Autodesk Inventor part; units mm, degrees
(part 4 of 4)
  line L912 (65.6705, -8.3885) -> (64.6705, -6.6564) projected
  line L913 (64.6705, -6.6564) -> (65.6705, -4.9244) projected
  line L914 (65.6705, -4.9244) -> (67.6705, -4.9244) projected
  line L915 (67.6705, -4.9244) -> (68.6705, -6.6564) projected
  line L916 (68.6705, -6.6564) -> (67.6705, -8.3885) projected
  line L917 (67.6705, -8.3885) -> (65.6705, -8.3885) projected
  line L918 (60.9385, -5.6564) -> (59.9385, -3.9244) projected
  line L919 (59.9385, -3.9244) -> (60.9385, -2.1923) projected
  line L920 (60.9385, -2.1923) -> (62.9385, -2.1923) projected
  line L921 (62.9385, -2.1923) -> (63.9385, -3.9244) projected
  line L922 (63.9385, -3.9244) -> (62.9385, -5.6564) projected
  line L923 (62.9385, -5.6564) -> (60.9385, -5.6564) projected
  line L924 (56.2064, -8.3885) -> (55.2064, -6.6564) projected
  line L925 (55.2064, -6.6564) -> (56.2064, -4.9244) projected
  line L926 (56.2064, -4.9244) -> (58.2064, -4.9244) projected
  line L927 (58.2064, -4.9244) -> (59.2064, -6.6564) projected
  line L928 (59.2064, -6.6564) -> (58.2064, -8.3885) projected
  line L929 (58.2064, -8.3885) -> (56.2064, -8.3885) projected
  line L930 (51.4744, -5.6564) -> (50.4744, -3.9244) projected
  line L931 (50.4744, -3.9244) -> (51.4744, -2.1923) projected
  line L932 (51.4744, -2.1923) -> (53.4744, -2.1923) projected
  line L933 (53.4744, -2.1923) -> (54.4744, -3.9244) projected
  line L934 (54.4744, -3.9244) -> (53.4744, -5.6564) projected
  line L935 (53.4744, -5.6564) -> (51.4744, -5.6564) projected
  line L936 (46.7423, -8.3885) -> (45.7423, -6.6564) projected
  line L937 (45.7423, -6.6564) -> (46.7423, -4.9244) projected
  line L938 (46.7423, -4.9244) -> (48.7423, -4.9244) projected
  line L939 (48.7423, -4.9244) -> (49.7423, -6.6564) projected
  line L940 (49.7423, -6.6564) -> (48.7423, -8.3885) projected
  line L941 (48.7423, -8.3885) -> (46.7423, -8.3885) projected
  line L942 (42.0103, -5.6564) -> (41.0103, -3.9244) projected
  line L943 (41.0103, -3.9244) -> (42.0103, -2.1923) projected
  line L944 (42.0103, -2.1923) -> (44.0103, -2.1923) projected
  line L945 (44.0103, -2.1923) -> (45.0103, -3.9244) projected
  line L946 (45.0103, -3.9244) -> (44.0103, -5.6564) projected
  line L947 (44.0103, -5.6564) -> (42.0103, -5.6564) projected
  line L948 (37.2782, -8.3885) -> (36.2782, -6.6564) projected
  line L949 (36.2782, -6.6564) -> (37.2782, -4.9244) projected
  line L950 (37.2782, -4.9244) -> (39.2782, -4.9244) projected
  line L951 (39.2782, -4.9244) -> (40.2782, -6.6564) projected
  line L952 (40.2782, -6.6564) -> (39.2782, -8.3885) projected
  line L953 (39.2782, -8.3885) -> (37.2782, -8.3885) projected
  line L954 (32.5462, -5.6564) -> (31.5462, -3.9244) projected
  line L955 (31.5462, -3.9244) -> (32.5462, -2.1923) projected
  line L956 (32.5462, -2.1923) -> (34.5462, -2.1923) projected
  line L957 (34.5462, -2.1923) -> (35.5462, -3.9244) projected
  line L958 (35.5462, -3.9244) -> (34.5462, -5.6564) projected
  line L959 (34.5462, -5.6564) -> (32.5462, -5.6564) projected
  line L960 (27.8141, -8.3885) -> (26.8141, -6.6564) projected
  line L961 (26.8141, -6.6564) -> (27.8141, -4.9244) projected
  line L962 (27.8141, -4.9244) -> (29.8141, -4.9244) projected
  line L963 (29.8141, -4.9244) -> (30.8141, -6.6564) projected
  line L964 (30.8141, -6.6564) -> (29.8141, -8.3885) projected
  line L965 (29.8141, -8.3885) -> (27.8141, -8.3885) projected
  line L966 (23.0821, -5.6564) -> (22.0821, -3.9244) projected
  line L967 (22.0821, -3.9244) -> (23.0821, -2.1923) projected
  line L968 (23.0821, -2.1923) -> (25.0821, -2.1923) projected
  line L969 (25.0821, -2.1923) -> (26.0821, -3.9244) projected
  line L970 (26.0821, -3.9244) -> (25.0821, -5.6564) projected
  line L971 (25.0821, -5.6564) -> (23.0821, -5.6564) projected
  line L972 (75.1346, -2.9244) -> (74.1346, -1.1923) projected
  line L973 (74.1346, -1.1923) -> (75.1346, 0.5397) projected
  line L974 (75.1346, 0.5397) -> (77.1346, 0.5397) projected
  line L975 (77.1346, 0.5397) -> (78.1346, -1.1923) projected
  line L976 (78.1346, -1.1923) -> (77.1346, -2.9244) projected
  line L977 (77.1346, -2.9244) -> (75.1346, -2.9244) projected
  line L978 (70.4026, -0.1923) -> (69.4026, 1.5397) projected
  line L979 (69.4026, 1.5397) -> (70.4026, 3.2718) projected
  line L980 (70.4026, 3.2718) -> (72.4026, 3.2718) projected
  line L981 (72.4026, 3.2718) -> (73.4026, 1.5397) projected
  line L982 (73.4026, 1.5397) -> (72.4026, -0.1923) projected
  line L983 (72.4026, -0.1923) -> (70.4026, -0.1923) projected
  line L984 (65.6705, -2.9244) -> (64.6705, -1.1923) projected
  line L985 (64.6705, -1.1923) -> (65.6705, 0.5397) projected
  line L986 (65.6705, 0.5397) -> (67.6705, 0.5397) projected
  line L987 (67.6705, 0.5397) -> (68.6705, -1.1923) projected
  line L988 (68.6705, -1.1923) -> (67.6705, -2.9244) projected
  line L989 (67.6705, -2.9244) -> (65.6705, -2.9244) projected
  line L990 (60.9385, -0.1923) -> (59.9385, 1.5397) projected
  line L991 (59.9385, 1.5397) -> (60.9385, 3.2718) projected
  line L992 (60.9385, 3.2718) -> (62.9385, 3.2718) projected
  line L993 (62.9385, 3.2718) -> (63.9385, 1.5397) projected
  line L994 (63.9385, 1.5397) -> (62.9385, -0.1923) projected
  line L995 (62.9385, -0.1923) -> (60.9385, -0.1923) projected
  line L996 (56.2064, -2.9244) -> (55.2064, -1.1923) projected
  line L997 (55.2064, -1.1923) -> (56.2064, 0.5397) projected
  line L998 (56.2064, 0.5397) -> (58.2064, 0.5397) projected
  line L999 (58.2064, 0.5397) -> (59.2064, -1.1923) projected
  line L1000 (59.2064, -1.1923) -> (58.2064, -2.9244) projected
  line L1001 (58.2064, -2.9244) -> (56.2064, -2.9244) projected
  line L1002 (51.4744, -0.1923) -> (50.4744, 1.5397) projected
  line L1003 (50.4744, 1.5397) -> (51.4744, 3.2718) projected
  line L1004 (51.4744, 3.2718) -> (53.4744, 3.2718) projected
  line L1005 (53.4744, 3.2718) -> (54.4744, 1.5397) projected
  line L1006 (54.4744, 1.5397) -> (53.4744, -0.1923) projected
  line L1007 (53.4744, -0.1923) -> (51.4744, -0.1923) projected
  line L1008 (46.7423, -2.9244) -> (45.7423, -1.1923) projected
  line L1009 (45.7423, -1.1923) -> (46.7423, 0.5397) projected
  line L1010 (46.7423, 0.5397) -> (48.7423, 0.5397) projected
  line L1011 (48.7423, 0.5397) -> (49.7423, -1.1923) projected
  line L1012 (49.7423, -1.1923) -> (48.7423, -2.9244) projected
  line L1013 (48.7423, -2.9244) -> (46.7423, -2.9244) projected
  line L1014 (42.0103, -0.1923) -> (41.0103, 1.5397) projected
  line L1015 (41.0103, 1.5397) -> (42.0103, 3.2718) projected
  line L1016 (42.0103, 3.2718) -> (44.0103, 3.2718) projected
  line L1017 (44.0103, 3.2718) -> (45.0103, 1.5397) projected
  line L1018 (45.0103, 1.5397) -> (44.0103, -0.1923) projected
  line L1019 (44.0103, -0.1923) -> (42.0103, -0.1923) projected
  line L1020 (37.2782, -2.9244) -> (36.2782, -1.1923) projected
  line L1021 (36.2782, -1.1923) -> (37.2782, 0.5397) projected
  line L1022 (37.2782, 0.5397) -> (39.2782, 0.5397) projected
  line L1023 (39.2782, 0.5397) -> (40.2782, -1.1923) projected
  line L1024 (40.2782, -1.1923) -> (39.2782, -2.9244) projected
  line L1025 (39.2782, -2.9244) -> (37.2782, -2.9244) projected
  line L1026 (32.5462, -0.1923) -> (31.5462, 1.5397) projected
  line L1027 (31.5462, 1.5397) -> (32.5462, 3.2718) projected
  line L1028 (32.5462, 3.2718) -> (34.5462, 3.2718) projected
  line L1029 (34.5462, 3.2718) -> (35.5462, 1.5397) projected
  line L1030 (35.5462, 1.5397) -> (34.5462, -0.1923) projected
  line L1031 (34.5462, -0.1923) -> (32.5462, -0.1923) projected
  line L1032 (27.8141, -2.9244) -> (26.8141, -1.1923) projected
  line L1033 (26.8141, -1.1923) -> (27.8141, 0.5397) projected
  line L1034 (27.8141, 0.5397) -> (29.8141, 0.5397) projected
  line L1035 (29.8141, 0.5397) -> (30.8141, -1.1923) projected
  line L1036 (30.8141, -1.1923) -> (29.8141, -2.9244) projected
  line L1037 (29.8141, -2.9244) -> (27.8141, -2.9244) projected
  line L1038 (23.0821, -0.1923) -> (22.0821, 1.5397) projected
  line L1039 (22.0821, 1.5397) -> (23.0821, 3.2718) projected
  line L1040 (23.0821, 3.2718) -> (25.0821, 3.2718) projected
  line L1041 (25.0821, 3.2718) -> (26.0821, 1.5397) projected
  line L1042 (26.0821, 1.5397) -> (25.0821, -0.1923) projected
  line L1043 (25.0821, -0.1923) -> (23.0821, -0.1923) projected
  line L1044 (75.1346, 2.5397) -> (74.1346, 4.2718) projected
  line L1045 (74.1346, 4.2718) -> (75.1346, 6.0038) projected
  line L1046 (75.1346, 6.0038) -> (77.1346, 6.0038) projected
  line L1047 (77.1346, 6.0038) -> (78.1346, 4.2718) projected
  line L1048 (78.1346, 4.2718) -> (77.1346, 2.5397) projected
  line L1049 (77.1346, 2.5397) -> (75.1346, 2.5397) projected
  line L1050 (70.4026, 5.2718) -> (69.4026, 7.0038) projected
  line L1051 (69.4026, 7.0038) -> (70.4026, 8.7359) projected
  line L1052 (70.4026, 8.7359) -> (72.4026, 8.7359) projected
  line L1053 (72.4026, 8.7359) -> (73.4026, 7.0038) projected
  line L1054 (73.4026, 7.0038) -> (72.4026, 5.2718) projected
  line L1055 (72.4026, 5.2718) -> (70.4026, 5.2718) projected
  line L1056 (65.6705, 2.5397) -> (64.6705, 4.2718) projected
  line L1057 (64.6705, 4.2718) -> (65.6705, 6.0038) projected
  line L1058 (65.6705, 6.0038) -> (67.6705, 6.0038) projected
  line L1059 (67.6705, 6.0038) -> (68.6705, 4.2718) projected
  line L1060 (68.6705, 4.2718) -> (67.6705, 2.5397) projected
  line L1061 (67.6705, 2.5397) -> (65.6705, 2.5397) projected
  line L1062 (60.9385, 5.2718) -> (59.9385, 7.0038) projected
  line L1063 (59.9385, 7.0038) -> (60.9385, 8.7359) projected
  line L1064 (60.9385, 8.7359) -> (62.9385, 8.7359) projected
  line L1065 (62.9385, 8.7359) -> (63.9385, 7.0038) projected
  line L1066 (63.9385, 7.0038) -> (62.9385, 5.2718) projected
  line L1067 (62.9385, 5.2718) -> (60.9385, 5.2718) projected
  line L1068 (56.2064, 2.5397) -> (55.2064, 4.2718) projected
  line L1069 (55.2064, 4.2718) -> (56.2064, 6.0038) projected
  line L1070 (56.2064, 6.0038) -> (58.2064, 6.0038) projected
  line L1071 (58.2064, 6.0038) -> (59.2064, 4.2718) projected
  line L1072 (59.2064, 4.2718) -> (58.2064, 2.5397) projected
  line L1073 (58.2064, 2.5397) -> (56.2064, 2.5397) projected
  line L1074 (51.4744, 5.2718) -> (50.4744, 7.0038) projected
  line L1075 (50.4744, 7.0038) -> (51.4744, 8.7359) projected
  line L1076 (51.4744, 8.7359) -> (53.4744, 8.7359) projected
  line L1077 (53.4744, 8.7359) -> (54.4744, 7.0038) projected
  line L1078 (54.4744, 7.0038) -> (53.4744, 5.2718) projected
  line L1079 (53.4744, 5.2718) -> (51.4744, 5.2718) projected
  line L1080 (46.7423, 2.5397) -> (45.7423, 4.2718) projected
  line L1081 (45.7423, 4.2718) -> (46.7423, 6.0038) projected
  line L1082 (46.7423, 6.0038) -> (48.7423, 6.0038) projected
  line L1083 (48.7423, 6.0038) -> (49.7423, 4.2718) projected
  line L1084 (49.7423, 4.2718) -> (48.7423, 2.5397) projected
  line L1085 (48.7423, 2.5397) -> (46.7423, 2.5397) projected
  line L1086 (42.0103, 5.2718) -> (41.0103, 7.0038) projected
  line L1087 (41.0103, 7.0038) -> (42.0103, 8.7359) projected
  line L1088 (42.0103, 8.7359) -> (44.0103, 8.7359) projected
  line L1089 (44.0103, 8.7359) -> (45.0103, 7.0038) projected
  line L1090 (45.0103, 7.0038) -> (44.0103, 5.2718) projected
  line L1091 (44.0103, 5.2718) -> (42.0103, 5.2718) projected
  line L1092 (37.2782, 2.5397) -> (36.2782, 4.2718) projected
  line L1093 (36.2782, 4.2718) -> (37.2782, 6.0038) projected
  line L1094 (37.2782, 6.0038) -> (39.2782, 6.0038) projected
  line L1095 (39.2782, 6.0038) -> (40.2782, 4.2718) projected
  line L1096 (40.2782, 4.2718) -> (39.2782, 2.5397) projected
  line L1097 (39.2782, 2.5397) -> (37.2782, 2.5397) projected
  line L1098 (32.5462, 5.2718) -> (31.5462, 7.0038) projected
  line L1099 (31.5462, 7.0038) -> (32.5462, 8.7359) projected
  line L1100 (32.5462, 8.7359) -> (34.5462, 8.7359) projected
  line L1101 (34.5462, 8.7359) -> (35.5462, 7.0038) projected
  line L1102 (35.5462, 7.0038) -> (34.5462, 5.2718) projected
  line L1103 (34.5462, 5.2718) -> (32.5462, 5.2718) projected
  line L1104 (27.8141, 2.5397) -> (26.8141, 4.2718) projected
  line L1105 (26.8141, 4.2718) -> (27.8141, 6.0038) projected
  line L1106 (27.8141, 6.0038) -> (29.8141, 6.0038) projected
  line L1107 (29.8141, 6.0038) -> (30.8141, 4.2718) projected
  line L1108 (30.8141, 4.2718) -> (29.8141, 2.5397) projected
  line L1109 (29.8141, 2.5397) -> (27.8141, 2.5397) projected
  line L1110 (23.0821, 5.2718) -> (22.0821, 7.0038) projected
  line L1111 (22.0821, 7.0038) -> (23.0821, 8.7359) projected
  line L1112 (23.0821, 8.7359) -> (25.0821, 8.7359) projected
  line L1113 (25.0821, 8.7359) -> (26.0821, 7.0038) projected
  line L1114 (26.0821, 7.0038) -> (25.0821, 5.2718) projected
  line L1115 (25.0821, 5.2718) -> (23.0821, 5.2718) projected
  line L1116 (75.1346, 8.0038) -> (74.1346, 9.7359) projected
  line L1117 (74.1346, 9.7359) -> (75.1346, 11.4679) projected
  line L1118 (75.1346, 11.4679) -> (77.1346, 11.4679) projected
  line L1119 (77.1346, 11.4679) -> (78.1346, 9.7359) projected
  line L1120 (78.1346, 9.7359) -> (77.1346, 8.0038) projected
  line L1121 (77.1346, 8.0038) -> (75.1346, 8.0038) projected
  line L1122 (65.6705, 8.0038) -> (64.6705, 9.7359) projected
  line L1123 (64.6705, 9.7359) -> (65.6705, 11.4679) projected
  line L1124 (65.6705, 11.4679) -> (67.6705, 11.4679) projected
  line L1125 (67.6705, 11.4679) -> (68.6705, 9.7359) projected
  line L1126 (68.6705, 9.7359) -> (67.6705, 8.0038) projected
  line L1127 (67.6705, 8.0038) -> (65.6705, 8.0038) projected
  line L1128 (56.2064, 8.0038) -> (55.2064, 9.7359) projected
  line L1129 (55.2064, 9.7359) -> (56.2064, 11.4679) projected
  line L1130 (56.2064, 11.4679) -> (58.2064, 11.4679) projected
  line L1131 (58.2064, 11.4679) -> (59.2064, 9.7359) projected
  line L1132 (59.2064, 9.7359) -> (58.2064, 8.0038) projected
  line L1133 (58.2064, 8.0038) -> (56.2064, 8.0038) projected
  line L1134 (46.7423, 8.0038) -> (45.7423, 9.7359) projected
  line L1135 (45.7423, 9.7359) -> (46.7423, 11.4679) projected
  line L1136 (46.7423, 11.4679) -> (48.7423, 11.4679) projected
  line L1137 (48.7423, 11.4679) -> (49.7423, 9.7359) projected
  line L1138 (49.7423, 9.7359) -> (48.7423, 8.0038) projected
  line L1139 (48.7423, 8.0038) -> (46.7423, 8.0038) projected
  line L1140 (37.2782, 8.0038) -> (36.2782, 9.7359) projected
  line L1141 (36.2782, 9.7359) -> (37.2782, 11.4679) projected
  line L1142 (37.2782, 11.4679) -> (39.2782, 11.4679) projected
  line L1143 (39.2782, 11.4679) -> (40.2782, 9.7359) projected
  line L1144 (40.2782, 9.7359) -> (39.2782, 8.0038) projected
  line L1145 (39.2782, 8.0038) -> (37.2782, 8.0038) projected
  line L1146 (27.8141, 8.0038) -> (26.8141, 9.7359) projected
  line L1147 (26.8141, 9.7359) -> (27.8141, 11.4679) projected
  line L1148 (27.8141, 11.4679) -> (29.8141, 11.4679) projected
  line L1149 (29.8141, 11.4679) -> (30.8141, 9.7359) projected
  line L1150 (30.8141, 9.7359) -> (29.8141, 8.0038) projected
  line L1151 (29.8141, 8.0038) -> (27.8141, 8.0038) projected
  line L1152 (-16.85, 17.7) -> (83.15, 17.7) projected
  line L1153 (-16.85, 17.7) -> (-16.85, -82.3) projected
  line L1154 (-16.85, -82.3) -> (83.15, -82.3) projected
  line L1155 (83.15, -82.3) -> (83.15, 17.7) projected
  line L1156 (16.85, -14) -> (16.85, -77.3) projected
  line L1157 (16.85, -77.3) -> (-11.85, -77.3) projected
  line L1158 (-11.85, -77.3) -> (-11.85, -14) projected
  line L1159 (4.5764, -14) -> (-11.85, -14) projected
  line L1160 (4.5764, -10.9307) -> (4.5764, -14) projected
  arc A0 (-8.8806, 7.8458) -> (4.5764, -10.9307) centre (0, 0) ccw projected
  arc A1 (-8.8806, 7.8458) -> (-9.068, 8.2614) centre (-9.068, 8.0114) ccw projected
  line L1161 (-9.25, 8.2614) -> (-9.068, 8.2614) projected
  line L1162 (-10, 9.0114) -> (-9.25, 8.2614) projected
  line L1163 (-10, 12.7) -> (-10, 9.0114) projected
  line L1164 (10, 12.7) -> (-10, 12.7) projected
  line L1165 (10, 9.0114) -> (10, 12.7) projected
  line L1166 (9.25, 8.2614) -> (10, 9.0114) projected
  line L1167 (9.068, 8.2614) -> (9.25, 8.2614) projected
  arc A2 (9.068, 8.2614) -> (8.8806, 7.8458) centre (9.068, 8.0114) ccw projected
  arc A3 (11.5236, -2.7619) -> (8.8806, 7.8458) centre (0, 0) ccw projected
  line L1168 (11.5236, -14) -> (11.5236, -2.7619) projected
  line L1169 (16.85, -14) -> (11.5236, -14) projected
  line L1170 (-16.85, 17.7) -> (83.15, 17.7)
  line L1171 (83.15, 17.7) -> (83.15, 12.7)
  line L1172 (83.15, 12.7) -> (-16.85, 12.7)
  line L1173 (-16.85, 12.7) -> (-16.85, 17.7)
  line L1174 (-16.85, -82.3) -> (-11.85, -82.3)
  line L1175 (-11.85, -82.3) -> (-11.85, 12.7)
  line L1176 (-11.85, 12.7) -> (-16.85, 12.7)
  line L1177 (-16.85, 12.7) -> (-16.85, -82.3)
  line L1178 (83.15, -82.3) -> (-11.85, -82.3)
  line L1179 (-11.85, -82.3) -> (-11.85, -77.3)
  line L1180 (-11.85, -77.3) -> (83.15, -77.3)
  line L1181 (83.15, -77.3) -> (83.15, -82.3)
  line L1182 (83.15, -77.3) -> (78.15, -77.3)
  line L1183 (78.15, -77.3) -> (78.15, 12.7)
  line L1184 (78.15, 12.7) -> (83.15, 12.7)
  line L1185 (83.15, 12.7) -> (83.15, -77.3)
  line L1186 (16.85, -77.3) -> (21.85, -77.3)
  line L1187 (21.85, -77.3) -> (21.85, 12.7)
  line L1188 (21.85, 12.7) -> (16.85, 12.7)
  line L1189 (16.85, 12.7) -> (16.85, -77.3)
  line L1190 (-14.35, 15.2) -> (80.65, 15.2) construction
  line L1191 (-14.35, 14.2) -> (80.65, 14.2)
  line L1192 (80.65, 16.2) -> (-14.35, 16.2)
  arc A4 (-14.35, 16.2) -> (-14.35, 14.2) centre (-14.35, 15.2) ccw
  arc A5 (80.65, 14.2) -> (80.65, 16.2) centre (80.65, 15.2) ccw
  line L1193 (80.65, 15.2) -> (80.65, -79.8) construction
  line L1194 (79.65, 15.2) -> (79.65, -79.8)
  line L1195 (81.65, -79.8) -> (81.65, 15.2)
  arc A6 (81.65, 15.2) -> (79.65, 15.2) centre (80.65, 15.2) ccw
  arc A7 (79.65, -79.8) -> (81.65, -79.8) centre (80.65, -79.8) ccw
  line L1196 (80.65, -79.8) -> (-14.35, -79.8) construction
  line L1197 (80.65, -80.8) -> (-14.35, -80.8)
  line L1198 (-14.35, -78.8) -> (80.65, -78.8)
  arc A8 (80.65, -80.8) -> (80.65, -78.8) centre (80.65, -79.8) ccw
  arc A9 (-14.35, -78.8) -> (-14.35, -80.8) centre (-14.35, -79.8) ccw
  line L1199 (-14.35, -79.8) -> (-14.35, 15.2) construction
  line L1200 (-13.35, -79.8) -> (-13.35, 15.2)
  line L1201 (-15.35, 15.2) -> (-15.35, -79.8)
  arc A10 (-15.35, -79.8) -> (-13.35, -79.8) centre (-14.35, -79.8) ccw
  arc A11 (-13.35, 15.2) -> (-15.35, 15.2) centre (-14.35, 15.2) ccw
  line L1202 (19.35, 15.2) -> (19.35, -79.8) construction
  line L1203 (18.35, 15.2) -> (18.35, -79.8)
  line L1204 (20.35, -79.8) -> (20.35, 15.2)
  arc A12 (20.35, 15.2) -> (18.35, 15.2) centre (19.35, 15.2) ccw
  arc A13 (18.35, -79.8) -> (20.35, -79.8) centre (19.35, -79.8) ccw
  point P0 (33.15, 15.2)
  point P1 (80.65, -32.3)
  point P2 (33.15, -79.8)
  point P3 (-14.35, -32.3)
  point P4 (19.35, -32.3)
  point P5 (81.65, 15.2)
  point P6 (-15.35, 15.2)
  point P7 (-15.35, -79.8)
  point P8 (-13.35, 14.2)
  point P9 (18.35, 14.2)
  point P10 (18.35, -78.8)
  point P11 (-13.35, -78.8)
  point P12 (79.65, -78.8)
  point P13 (20.35, -78.8)
  point P14 (20.35, 14.2)
  point P15 (79.65, 14.2)
  dimension "d65" = 5
  dimension "d66" = 5
  dimension "d67" = 5
  dimension "d69" = 1.5
  dimension "d70" = 1.5
  dimension "d71" = 1.5
  dimension "d72" = 1.5
  dimension "d73" = 1.5
  dimension "d74" = 1.5
  dimension "d75" = 1.5
  dimension "d76" = 1.5
  constraints: 80 end point, 22 tangent, 20 point on circle, 16 parallel, 10 centre point, 10 point on line, 8 perpendicular, 6 horizontal, 5 midpoint
  measures "d65" distance between parallel lines of L1170 L1172
  measures "d66" distance between parallel lines of L1189 L1187
  measures "d67" distance between parallel lines of L1185 L1183
  measures "d69" distance between parallel lines of L1158 L1200
  measures "d70" distance between parallel lines of L1153 L1201
  measures "d71" distance between parallel lines of L1178 L1197
  measures "d72" distance between parallel lines of L1157 L1198
  measures "d73" distance between parallel lines of L1185 L1195
  measures "d74" distance between parallel lines of L1191 L1172
  measures "d75" distance between parallel lines of L1187 L1204
  measures "d76" distance between parallel lines of L1189 L1203
extrude "Extrusion5" cut sketch "Sketch8" against normal blind 2 contours L1201 A4 L1191 L1200 L1172 | L1172 L1200 L1198 A9 L1201 | L1195 L1180 L1194 L1172 | L1172 L1194 L1191 A5 L1195 | A4 A11 L1200 L1191 | A9 L1198 L1200 A10 | L1195 A8 L1198 L1194 L1180 | A5 L1191 L1194 A6 | L1197 A10 L1200 L1198 L1175 | L1175 L1198 L1203 A13 L1197 | L1200 A11 L1192 A12 L1203 L1191 | A7 L1194 L1198 A8 | L1191 L1204 A12 L1192 A6 L1194 | A13 L1204 L1198 L1194 A7 L1197 | A13 L1203 L1198 L1204 | L1203 A12 L1204 L1191 | L1191 L1204 L1172 L1203 | L1203 L1180 L1204 L1198 | L1172 L1204 L1180 L1203
sketch "Sketch9" plane through (0, 0, 0) normal (0, -1, 0) x (1, 0, 0)
  arc A0 (81.65, 15.2) -> (80.65, 16.2) centre (80.65, 15.2) ccw projected
  line L0 (-14.35, 16.2) -> (80.65, 16.2) projected
  arc A1 (-14.35, 16.2) -> (-15.35, 15.2) centre (-14.35, 15.2) ccw projected
  line L1 (-15.35, -79.8) -> (-15.35, 15.2) projected
  arc A2 (-15.35, -79.8) -> (-14.35, -80.8) centre (-14.35, -79.8) ccw projected
  line L2 (80.65, -80.8) -> (-14.35, -80.8) projected
  arc A3 (80.65, -80.8) -> (81.65, -79.8) centre (80.65, -79.8) ccw projected
  line L3 (81.65, 15.2) -> (81.65, -79.8) projected
  line L4 (18.35, 14.2) -> (-13.35, 14.2) projected
  line L5 (18.35, -78.8) -> (18.35, 14.2) projected
  line L6 (-13.35, -78.8) -> (18.35, -78.8) projected
  line L7 (-13.35, 14.2) -> (-13.35, -78.8) projected
  line L8 (79.65, -78.8) -> (79.65, 14.2) projected
  line L9 (20.35, -78.8) -> (79.65, -78.8) projected
  line L10 (20.35, 14.2) -> (20.35, -78.8) projected
  line L11 (79.65, 14.2) -> (20.35, 14.2) projected
  point P0 (0, 0)
equation "\"d10\" = d9"
equation "\"d30\" = d29"
equation "\"d32\" = d31"
equation "\"d33\" = d29"
equation "\"d34\" = d33"
equation "\"d35\" = d29"
equation "\"d50\" = d45"
equation "\"d51\" = d50"
equation "\"d52\" = d50"
equation "\"d53\" = d52"
equation "\"d57\" = d47"
equation "\"d60\" = d54"
equation "\"d41\" = 0.5 * d40"
equation "\"d42\" = d41"
body "Solid1"
